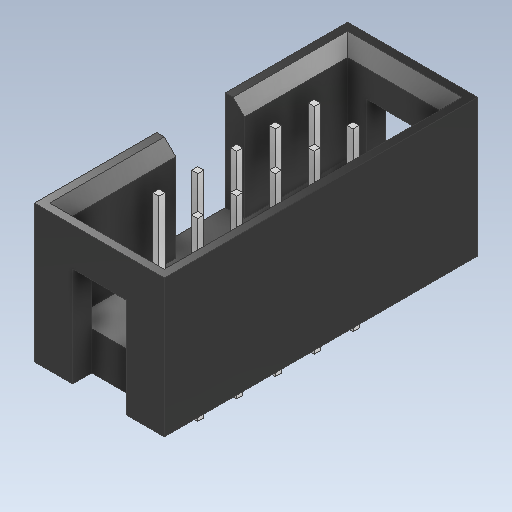
# Autodesk Inventor part: IDC_8_pin_connector
Saved by Autodesk Inventor 2020 (Build 240168000, 168)
## iProperties
Created: 2019-12-29
Part Number: IDC_8_pin_connector
Material: Generic
Document SubType Name: Modeling
Designer: ermoz
Density: 1 g/cm^3
Appearance: Default
Mass: 0.774416 g
Surface Area: 13.2201 cm^2
Volume: 0.774416 cm^3
Author: ermoz
Autodesk Inventor part; units mm, degrees
ref_plane "YZ Plane" through (0, 0, 0) normal (1, 0, 0) x (0, 1, 0)
ref_plane "XZ Plane" through (0, 0, 0) normal (0, 1, 0) x (-1, 0, 0)
ref_plane "XY Plane" through (0, 0, 0) normal (0, 0, 1) x (1, 0, 0)
sketch "Sketch1" plane through (0, 0, 0) normal (0, 1, 0) x (-1, 0, 0)
  line L0 (-4.25, 10.25) -> (4.25, 10.25)
  line L1 (4.25, 10.25) -> (4.25, -10.25)
  line L2 (4.25, -10.25) -> (-4.25, -10.25)
  line L3 (-4.25, -10.25) -> (-4.25, 10.25)
  line L4 (-4.25, 10.25) -> (4.25, -10.25) construction
  line L5 (4.25, 10.25) -> (-4.25, -10.25) construction
  point P0 (0, 0)
  dimension "d0" = 8.5
  dimension "d1" = 20.5
  constraints: 12 end point, 2 midpoint, 2 parallel, 1 horizontal, 1 perpendicular
  measures "d0" distance of L1.end L2.end
  measures "d1" distance of L0.end L1.end
extrude "Extrusion1" add sketch "Sketch1" along normal blind 2.5
sketch "Sketch2" plane through (0, 2.5, 0) normal (0, 1, 0) x (1, 0, 0)
  line L0 (-4.25, -10.25) -> (4.25, -10.25) projected
  line L1 (4.25, -10.25) -> (4.25, 10.25) projected
  line L2 (-4.25, -10.25) -> (4.25, -10.25)
  line L3 (4.25, -10.25) -> (4.25, 10.25)
  line L4 (4.25, 10.25) -> (-4.25, 10.25)
  line L5 (-4.25, 10.25) -> (-4.25, -10.25)
  line L6 (-3, -9) -> (3, -9)
  line L7 (3, -9) -> (3, 9)
  line L8 (3, 9) -> (-3, 9)
  line L9 (-3, 9) -> (-3, -9)
  line L10 (-3, -9) -> (3, 9) construction
  line L11 (3, -9) -> (-3, 9) construction
  line L12 (-4.25, 10.25) -> (-4.25, -10.25) projected
  line L13 (-4.25, 0) -> (-3, 0)
  line L14 (-3, -2.25) -> (-4.25, -2.25)
  line L15 (-4.25, -2.25) -> (-4.25, 2.25)
  line L16 (-4.25, 2.25) -> (-3, 2.25)
  line L17 (-3, 2.25) -> (-3, -2.25)
  line L18 (-3, -2.25) -> (-4.25, 2.25) construction
  line L19 (-4.25, -2.25) -> (-3, 2.25) construction
  point P0 (0, 0)
  point P1 (-3.625, 0)
  dimension "d4" = 6
  dimension "d5" = 18
  dimension "d6" = 4.5
  constraints: 34 end point, 7 midpoint, 6 parallel, 3 horizontal, 3 perpendicular, 1 point on line
  measures "d4" distance of L8.end L7.end
  measures "d5" distance of L7.end L6.end
  measures "d6" distance of L14.end L15.end
extrude "Extrusion2" add sketch "Sketch2" along normal blind 6.5 contours L5 L14 L9 L6 L7 L8 L16 L4 L1 L0
sketch "Sketch3" plane through (-4.25, 0, 10.25) normal (0, 0, 1) x (1, 0, 0)
  line L0 (4.25, 0) -> (4.25, 3.25)
  line L1 (2.5, 0) -> (6, 0)
  line L2 (6, 0) -> (6, 6.5)
  line L3 (6, 6.5) -> (2.5, 6.5)
  line L4 (2.5, 6.5) -> (2.5, 0)
  line L5 (2.5, 0) -> (6, 6.5) construction
  line L6 (6, 0) -> (2.5, 6.5) construction
  dimension "d9" = 3.25
  dimension "d10" = 3.5
  dimension "d11" = 6.5
  constraints: 14 end point, 2 midpoint, 2 parallel, 1 horizontal, 1 perpendicular, 1 vertical
  measures "d9" distance of L0.start L0.end
  measures "d10" distance of L3.end L2.end
  measures "d11" distance of L2.end L1.end
extrude "Extrusion3" cut sketch "Sketch3" against normal blind 1.25
sketch "Sketch4" plane through (4.25, 0, -10.25) normal (0, 0, -1) x (-1, 0, 0)
  line L0 (4.25, 0) -> (4.25, 3.25)
  line L1 (2.5, 0) -> (6, 0)
  line L2 (6, 0) -> (6, 6.5)
  line L3 (6, 6.5) -> (2.5, 6.5)
  line L4 (2.5, 6.5) -> (2.5, 0)
  line L5 (2.5, 0) -> (6, 6.5) construction
  line L6 (6, 0) -> (2.5, 6.5) construction
  dimension "d14" = 3.25
  dimension "d15" = 3.5
  dimension "d16" = 6.5
  constraints: 14 end point, 2 midpoint, 2 parallel, 1 horizontal, 1 perpendicular, 1 vertical
  measures "d14" distance of L0.start L0.end
  measures "d15" distance of L3.end L2.end
  measures "d16" distance of L2.end L1.end
extrude "Extrusion4" cut sketch "Sketch4" against normal blind 1.25
chamfer "Chamfer1" distance 0.75 angle 45 5 edges at (3, 9, 0) (0, 9, 9) (-3, 9, 5.625) (-3, 9, -5.625) (0, 9, -9)
sketch "Sketch5" plane through (0, 2.5, 0) normal (0, 1, 0) x (1, 0, 0)
  line L0 (1.27, 0) -> (-1.27, 0)
  line L1 (1.07, 5.28) -> (1.47, 5.28)
  line L2 (1.47, 5.28) -> (1.47, 4.88)
  line L3 (1.47, 4.88) -> (1.07, 4.88)
  line L4 (1.07, 4.88) -> (1.07, 5.28)
  line L5 (1.07, 5.28) -> (1.47, 4.88) construction
  line L6 (1.47, 5.28) -> (1.07, 4.88) construction
  line L7 (-1.07, 5.28) -> (-1.47, 5.28)
  line L8 (-1.47, 5.28) -> (-1.47, 4.88)
  line L9 (-1.47, 4.88) -> (-1.07, 4.88)
  line L10 (-1.07, 4.88) -> (-1.07, 5.28)
  line L11 (-1.07, 5.28) -> (-1.47, 4.88) construction
  line L12 (-1.47, 5.28) -> (-1.07, 4.88) construction
  line L13 (1.07, 2.74) -> (1.47, 2.74)
  line L14 (1.47, 2.74) -> (1.47, 2.34)
  line L15 (1.47, 2.34) -> (1.07, 2.34)
  line L16 (1.07, 2.34) -> (1.07, 2.74)
  line L17 (1.07, 2.74) -> (1.47, 2.34) construction
  line L18 (1.47, 2.74) -> (1.07, 2.34) construction
  line L19 (-1.07, 2.74) -> (-1.47, 2.74)
  line L20 (-1.47, 2.74) -> (-1.47, 2.34)
  line L21 (-1.47, 2.34) -> (-1.07, 2.34)
  line L22 (-1.07, 2.34) -> (-1.07, 2.74)
  line L23 (-1.07, 2.74) -> (-1.47, 2.34) construction
  line L24 (-1.47, 2.74) -> (-1.07, 2.34) construction
  line L25 (1.07, 0.2) -> (1.47, 0.2)
  line L26 (1.47, 0.2) -> (1.47, -0.2)
  line L27 (1.47, -0.2) -> (1.07, -0.2)
  line L28 (1.07, -0.2) -> (1.07, 0.2)
  line L29 (1.07, 0.2) -> (1.47, -0.2) construction
  line L30 (1.47, 0.2) -> (1.07, -0.2) construction
  line L31 (-1.07, 0.2) -> (-1.47, 0.2)
  line L32 (-1.47, 0.2) -> (-1.47, -0.2)
  line L33 (-1.47, -0.2) -> (-1.07, -0.2)
  line L34 (-1.07, -0.2) -> (-1.07, 0.2)
  line L35 (-1.07, 0.2) -> (-1.47, -0.2) construction
  line L36 (-1.47, 0.2) -> (-1.07, -0.2) construction
  line L37 (1.07, -5.28) -> (1.47, -5.28)
  line L38 (1.47, -5.28) -> (1.47, -4.88)
  line L39 (1.47, -4.88) -> (1.07, -4.88)
  line L40 (1.07, -4.88) -> (1.07, -5.28)
  line L41 (-1.07, -5.28) -> (-1.47, -5.28)
  line L42 (-1.47, -5.28) -> (-1.47, -4.88)
  line L43 (-1.47, -4.88) -> (-1.07, -4.88)
  line L44 (-1.07, -4.88) -> (-1.07, -5.28)
  line L45 (1.07, -2.74) -> (1.47, -2.74)
  line L46 (1.47, -2.74) -> (1.47, -2.34)
  line L47 (1.47, -2.34) -> (1.07, -2.34)
  line L48 (1.07, -2.34) -> (1.07, -2.74)
  line L49 (-1.07, -2.74) -> (-1.47, -2.74)
  line L50 (-1.47, -2.74) -> (-1.47, -2.34)
  line L51 (-1.47, -2.34) -> (-1.07, -2.34)
  line L52 (-1.07, -2.34) -> (-1.07, -2.74)
  point P0 (0, 0)
  dimension "d22" = 1.27
  dimension "d27" = 0.4
  dimension "d28" = 0.4
  dimension "d29" = 0.4
  dimension "d30" = 0.4
  dimension "d31" = 0.4
  dimension "d32" = 0.4
  dimension "d33" = 0.4
  dimension "d34" = 0.4
  dimension "d35" = 0.4
  dimension "d36" = 0.4
  constraints: 106 end point, 12 parallel, 7 horizontal, 6 perpendicular, 4 midpoint
  measures "d22" distance of point (0, 0) L0.start
  measures "d27" distance of L2.end L3.end
  measures "d28" distance of L1.end L2.end
  measures "d29" distance of L9.end L8.end
  measures "d30" distance of L8.end L7.end
  measures "d31" distance of L14.end L15.end
  measures "d32" distance of L13.end L14.end
  measures "d33" distance of L21.end L20.end
  measures "d34" distance of L20.end L19.end
  measures "d35" distance of L26.end L27.end
  measures "d36" distance of L25.end L26.end
extrude "Extrusion5" cut sketch "Sketch5" against normal blind 6
extrude "Extrusion6" add sketch "Sketch5" along normal blind 6 and the other way blind 5.5 separate body
body "Solid1"
body "Solid2"
